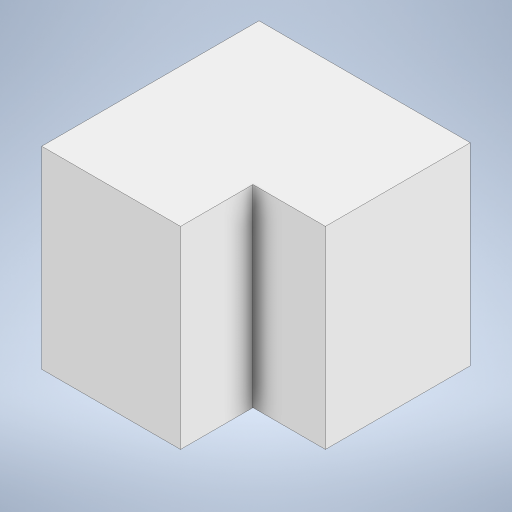
# Autodesk Inventor part: Corner_Cabinet
Saved by Autodesk Inventor 2024 (Build 280153000, 153)
## iProperties
Created: 2023-03-29
Part Number: Corner_Cabinet
Material: Wood (Birch)
Document SubType Name: Modeling
Designer: Tom
Density: 0.55 g/cm^3
Appearance: White
Author: Tom
Autodesk Inventor part; units mm, degrees
ref_plane "YZ Plane" through (0, 0, 0) normal (1, 0, 0) x (0, 1, 0)
ref_plane "XZ Plane" through (0, 0, 0) normal (0, 1, 0) x (-1, 0, 0)
ref_plane "XY Plane" through (0, 0, 0) normal (0, 0, 1) x (1, 0, 0)
sketch "Sketch1" plane through (0, 0, 0) normal (0, 1, 0) x (-1, 0, 0)
  line L0 (0, 0) -> (-889, 0)
  line L1 (-889, 0) -> (-889, 609.6)
  line L2 (-584.2, 914.4) -> (0, 914.4)
  line L3 (0, 914.4) -> (0, 0)
  line L4 (-584.2, 914.4) -> (-584.2, 609.6)
  line L5 (-584.2, 609.6) -> (-889, 609.6)
  dimension "d9" = 914.4
  dimension "d10" = 889
  dimension "d11" = 609.6
  dimension "d12" = 304.8
  dimension "d13" = 584.2
  constraints: 12 end point, 2 parallel, 1 horizontal, 1 perpendicular
  measures "d9" distance of L2.end L0.start
  measures "d10" distance of L0.start L0.end
  measures "d11" distance of L0.end L1.end
  measures "d12" distance of L4.end L1.end
  measures "d13" distance of L2.start L2.end
extrude "Extrusion1" add sketch "Sketch1" along normal blind 812.8
body "Solid1"
